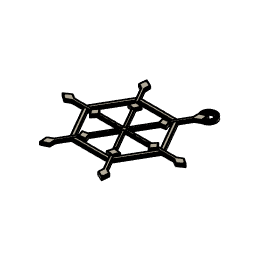
snowflake 4 (Autodesk Fusion 360 design; units mm, degrees)
Autodesk Fusion 360 part; units mm, degrees
note: some values were not read from the file. Chosen so that the rebuilt part matches the saved one: which bodies a step acts on.
(part 1 of 2)
sketch "Sketch1" plane through (0, 0, 0) normal (0, 0, 1) x (1, 0, 0)
  line L0 (-3.7004, 3.4114) -> (-1.9935, 3.4678)
  line L1 (-1.9935, 3.4678) -> (-1.0859, 4.9144)
  line L2 (-1.0859, 4.9144) -> (-2.4343, 6.3915)
  line L3 (-2.4343, 6.3915) -> (-20.127, 37.1684)
  line L4 (-20.127, 37.1684) -> (-21.9909, 36.0969)
  line L5 (-21.9909, 36.0969) -> (-4.2982, 5.32)
  line L6 (-4.2982, 5.32) -> (-3.7004, 3.4114)
  line L7 (-1.9935, 3.4678) -> (0, 0) construction
  dimension "d403" = 25
  dimension "d404" = 124
  dimension "d405" = 105.5
  dimension "d406" = 4
  dimension "d407" = 35.5
  dimension "d408" = 2.15
  dimension "d409" = 2
  dimension "d411" = 1.7068
  constraint coincident L7.end origin
  constraint symmetric L0 L1 L7
  constraint symmetric L2 L6 L7
  constraint symmetric L3 L5 L7
  constraint perpendicular L4 L5
  constraint perpendicular L3 L4
  measures "d403" angle of L2 L6
  measures "d404" angle of L0 L1
  measures "d405" angle of L1 L2
  measures "d406" distance of L0.end L7.end
  measures "d407" distance of L2.end L3.end
  measures "d408" distance of L3 L5
  measures "d409" distance of L1.end L2.end
  measures "d411" horizontal distance of L0.start L0.end
extrude "Extrude1" add sketch "Sketch1" along normal blind 5 makes body 1
pattern_circular "C-Pattern1" count 6 over 360 about axis through (0, 0, 1.75) along (0, 0, 1) of bodies 1 makes body 2 at (-18.5856, 1.1096, 1.6667) makes body 3 at (-14.3296, -26.8562, 1.6667) makes body 4 at (16.0934, -25.8379, 3.3333) makes body 5 at (18.5856, -1.1096, 1.6667) makes body 6 at (10.2538, 15.5408, 1.6667)
sketch "Sketch2" plane through (0, 0, 0) normal (0, 0, 1) x (1, 0, 0)
  line L0 (-31.5265, 40.9182) -> (-28.4205, 49.2257)
  line L1 (-28.4205, 49.2257) -> (-19.673, 47.7619)
  line L2 (-19.673, 47.7619) -> (-22.6772, 39.2781)
  line L3 (-22.6772, 39.2781) -> (-31.5265, 40.9182)
  line L4 (-28.4205, 49.2257) -> (-22.6772, 39.2781) construction
  line L5 (0, 1.75) -> (0, 22.5) construction
  line L6 (-20.127, 37.1684) -> (-21.9909, 36.0969) construction
  dimension "d416" = 30
  dimension "d417" = 3.1
  dimension "d418" = 99
  dimension "d419" = 80
  dimension "d420" = 9
  constraint coincident origin L4
  constraint symmetric L0 L1 L4
  constraint symmetric L2 L3 L4
  measures "d416" angle of L4 L5
  measures "d417" distance of L2.end L6
  measures "d418" angle of L2 L3
  measures "d419" angle of L1 L2
  measures "d420" distance of L1.end L2.end
extrude "Extrude2" add sketch "Sketch2" along normal up to surface (5 mm away) separate body makes body 7
pattern_circular "C-Pattern2" count 6 over 360 about axis through (0, 0, 1.75) along (0, 0, 1) of bodies 7 makes body 8 at (-51.1316, 2.2812, 0) makes body 9 at (-27.5414, -43.1407, 0) makes body 10 at (23.5902, -45.4219, 0) makes body 11 at (51.1316, -2.2812, 0) makes body 12 at (27.5414, 43.1407, 0)
sketch "Sketch3" plane through (0, 0, 0) normal (0, 0, 1) x (1, 0, 0)
  line L0 (-31.1618, 51.3738) -> (-29.6618, 51.3757)
  line L1 (-29.6618, 51.3757) -> (-28.9101, 52.6738)
  line L2 (-28.9101, 52.6738) -> (-43.4101, 77.7885)
  line L3 (-43.4101, 77.7885) -> (-43.4101, 86.9885)
  line L4 (-43.4101, 86.9885) -> (-50.3625, 90.2305)
  line L5 (-50.3625, 90.2305) -> (-52.9606, 88.7305)
  line L6 (-52.9606, 88.7305) -> (-53.6292, 81.0885)
  line L7 (-53.6292, 81.0885) -> (-45.6618, 76.4885)
  line L8 (-45.6618, 76.4885) -> (-31.1618, 51.3738)
  line L9 (-29.6618, 51.3757) -> (-51.6616, 89.4805) construction
  line L10 (0, 1.75) -> (0, 22.5) construction
  point P0 (-28.4205, 49.2257)
  dimension "d425" = 30
  dimension "d427" = 2.6
  dimension "d428" = 1.5
  dimension "d429" = 2.4826
  dimension "d430" = 60
  dimension "d431" = 70
  dimension "d432" = 3
  dimension "d433" = 9.2
  dimension "d434" = 29
  constraint midpoint L5 L9.end
  constraint coincident origin L9
  constraint symmetric L2 L8 L9
  constraint symmetric L0 L1 L9
  constraint symmetric L3 L7 L9
  constraint symmetric L4 L6 L9
  constraint perpendicular L5 L9
  constraint parallel L2 L8
  measures "d425" angle of L9 L10
  measures "d427" distance of L2 L8
  measures "d428" distance of L0.end L1.end
  measures "d429" distance of L0.end P0
  measures "d430" angle of L3 L7
  measures "d431" angle of L4 L6
  measures "d432" distance of L4.end L5.end
  measures "d433" distance of L2.end L3.end
  measures "d434" distance of L1.end L2.end
extrude "Extrude3" add sketch "Sketch3" along normal up to surface (5 mm away) separate body makes body 13
pattern_circular "C-Pattern3" count 6 over 360 about axis through (0, 0, 1.75) along (0, 0, 1) of bodies 13 makes body 14 at (-94.3835, 0.4333, 0) makes body 15 at (-47.567, -81.5218, 0) makes body 16 at (46.8165, -81.9552, 0) makes body 17 at (94.3835, -0.4333, 0) makes body 18 at (47.567, 81.5218, 0)
sketch "Sketch4" plane through (0, 0, 0) normal (0, 0, 1) x (1, 0, 0)
  line L0 (-3.7004, 3.4114) -> (-4.2982, 5.32)
  line L1 (-4.2982, 5.32) -> (-21.9909, 36.0969)
  line L2 (-21.9909, 36.0969) -> (-20.127, 37.1684)
  line L3 (-20.127, 37.1684) -> (-2.4343, 6.3915)
  line L4 (-2.4343, 6.3915) -> (-1.0859, 4.9144)
  line L5 (-1.0859, 4.9144) -> (-1.9935, 3.4678)
  line L6 (-1.9935, 3.4678) -> (-3.7004, 3.4114)
  line L7 (-19.673, 47.7619) -> (-22.6772, 39.2781)
  line L8 (-22.6772, 39.2781) -> (-31.5265, 40.9182)
  line L9 (-31.5265, 40.9182) -> (-28.4205, 49.2257)
  line L10 (-28.4205, 49.2257) -> (-19.673, 47.7619)
  line L11 (-31.1618, 51.3738) -> (-45.6618, 76.4885)
  line L12 (-45.6618, 76.4885) -> (-53.6292, 81.0885)
  line L13 (-53.6292, 81.0885) -> (-52.9606, 88.7305)
  line L14 (-52.9606, 88.7305) -> (-50.3625, 90.2305)
  line L15 (-50.3625, 90.2305) -> (-43.4101, 86.9885)
  line L16 (-43.4101, 86.9885) -> (-43.4101, 77.7885)
  line L17 (-43.4101, 77.7885) -> (-28.9101, 52.6738)
  line L18 (-28.9101, 52.6738) -> (-29.6618, 51.3757)
  line L19 (-29.6618, 51.3757) -> (-31.1618, 51.3738)
  line L20 (-19.5741, 39.2164) -> (-1.2157, 7.2815)
  line L21 (-1.2157, 7.2815) -> (0.791, 5.0833)
  line L22 (0.791, 5.0833) -> (-1.1469, 1.995)
  line L23 (-1.1469, 1.995) -> (-4.7908, 1.8745)
  line L24 (-4.7908, 1.8745) -> (-5.6805, 4.7148)
  line L25 (-5.6805, 4.7148) -> (-24.0389, 36.6497)
  line L26 (-24.0389, 36.6497) -> (-19.5741, 39.2164)
  line L27 (-33.5576, 39.7691) -> (-29.3924, 50.9092)
  line L28 (-29.3924, 50.9092) -> (-17.6623, 48.9462)
  line L29 (-17.6623, 48.9462) -> (-21.6909, 37.5697)
  line L30 (-21.6909, 37.5697) -> (-33.5576, 39.7691)
  line L31 (-28.7964, 49.8768) -> (-32.0271, 49.8726)
  line L32 (-32.0271, 49.8726) -> (-46.7598, 75.3904)
  line L33 (-46.7598, 75.3904) -> (-55.2068, 80.2673)
  line L34 (-55.2068, 80.2673) -> (-54.3868, 89.6391)
  line L35 (-54.3868, 89.6391) -> (-50.4363, 91.9199)
  line L36 (-50.4363, 91.9199) -> (-41.9101, 87.9441)
  line L37 (-41.9101, 87.9441) -> (-41.9101, 78.1904)
  line L38 (-41.9101, 78.1904) -> (-27.1774, 52.6726)
  line L39 (-27.1774, 52.6726) -> (-28.7964, 49.8768)
  line L40 (-54.3868, 89.6391) -> (-54.0403, 93.6005)
  line L41 (-54.0403, 93.6005) -> (-50.4363, 91.9199)
  line L42 (-27.1774, 52.6726) -> (-25.8135, 50.3103)
  line L43 (-32.0271, 49.8726) -> (-30.6632, 47.5103)
  line L44 (-19.5741, 39.2164) -> (-20.5232, 40.8673)
  line L45 (-24.0389, 36.6497) -> (-24.9109, 38.1665)
  dimension "d439" = -1.5
  dimension "d440" = -1.5
  dimension "d441" = -1.5
  constraint parallel L34 L40
  constraint collinear L36 L41
  constraint coincident L28 L42.end
  constraint parallel L38 L42
  constraint coincident L27 L43.end
  constraint parallel L32 L43
  constraint coincident L29 L44.end
  constraint perpendicular L26 L44
  constraint coincident L30 L45.end
  constraint perpendicular L26 L45
  measures "d441" distance of L19
extrude "Extrude4" add sketch "Sketch4" along normal up to surface (5 mm away) separate body makes body 19
pattern_circular "C-Pattern4" count 6 over 360 about axis through (0, 0, 1.75) along (0, 0, 1) of bodies 19 makes body 20 at (-105.9089, 0, 0) makes body 21 at (-52.9545, -91.7198, 0) makes body 22 at (52.9545, -91.7198, 0) makes body 23 at (105.9089, 0, 0) makes body 24 at (52.9545, 91.7198, 0)
combine "Combine1" operation add target body 19 tool bodies 21 24 22 23 20
sketch "Sketch5" plane through (0, 0, 0) normal (0, 0, 1) x (1, 0, 0)
  line L0 (-5.1366, 2.9784) -> (-5.6805, 4.7148)
  line L1 (-5.6805, 4.7148) -> (-24.9109, 38.1665)
  line L2 (-24.9109, 38.1665) -> (-33.5576, 39.7691)
  line L3 (-33.5576, 39.7691) -> (-30.6632, 47.5103)
  line L4 (-30.6632, 47.5103) -> (-46.7598, 75.3904)
  line L5 (-46.7598, 75.3904) -> (-55.2068, 80.2673)
  line L6 (-55.2068, 80.2673) -> (-54.0403, 93.6005)
  line L7 (-54.0403, 93.6005) -> (-41.9101, 87.9441)
  line L8 (-41.9101, 87.9441) -> (-41.9101, 78.1904)
  line L9 (-41.9101, 78.1904) -> (-25.8135, 50.3103)
  line L10 (-25.8135, 50.3103) -> (-17.6623, 48.9462)
  line L11 (-17.6623, 48.9462) -> (-20.5232, 40.8673)
  line L12 (-20.5232, 40.8673) -> (-1.2157, 7.2815)
  line L13 (-1.2157, 7.2815) -> (0.0111, 5.9377)
  line L14 (0.0111, 5.9377) -> (1.2429, 7.2769)
  line L15 (1.2429, 7.2769) -> (20.5977, 40.6567)
  line L16 (20.5977, 40.6567) -> (17.6623, 48.9462)
  line L17 (17.6623, 48.9462) -> (25.8135, 50.3103)
  line L18 (25.8135, 50.3103) -> (41.9101, 78.1904)
  line L19 (41.9101, 78.1904) -> (41.9101, 87.9441)
  line L20 (41.9101, 87.9441) -> (54.0403, 93.6005)
  line L21 (54.0403, 93.6005) -> (55.2068, 80.2673)
  line L22 (55.2068, 80.2673) -> (46.7598, 75.3904)
  line L23 (46.7598, 75.3904) -> (30.6632, 47.5103)
  line L24 (30.6632, 47.5103) -> (33.5576, 39.7691)
  line L25 (33.5576, 39.7691) -> (25.1306, 38.2072)
  line L26 (25.1306, 38.2072) -> (5.6981, 4.6936)
  line L27 (5.6981, 4.6936) -> (5.1477, 2.9592)
  line L28 (5.1477, 2.9592) -> (6.9234, 2.5621)
  line L29 (6.9234, 2.5621) -> (45.5086, 2.4902)
  line L30 (45.5086, 2.4902) -> (51.2198, 9.1772)
  line L31 (51.2198, 9.1772) -> (56.4767, 2.8)
  line L32 (56.4767, 2.8) -> (88.6699, 2.8)
  line L33 (88.6699, 2.8) -> (97.1169, 7.6768)
  line L34 (97.1169, 7.6768) -> (108.0805, 0)
  line L35 (108.0805, 0) -> (97.1169, -7.6768)
  line L36 (97.1169, -7.6768) -> (88.6699, -2.8)
  line L37 (88.6699, -2.8) -> (56.4767, -2.8)
  line L38 (56.4767, -2.8) -> (51.2198, -9.1772)
  line L39 (51.2198, -9.1772) -> (45.6537, -2.6601)
  line L40 (45.6537, -2.6601) -> (6.9138, -2.5879)
  line L41 (6.9138, -2.5879) -> (5.1366, -2.9784)
  line L42 (5.1366, -2.9784) -> (5.6805, -4.7148)
  line L43 (5.6805, -4.7148) -> (24.9109, -38.1665)
  line L44 (24.9109, -38.1665) -> (33.5576, -39.7691)
  line L45 (33.5576, -39.7691) -> (30.6632, -47.5103)
  line L46 (30.6632, -47.5103) -> (46.7598, -75.3904)
  line L47 (46.7598, -75.3904) -> (55.2068, -80.2673)
  line L48 (55.2068, -80.2673) -> (54.0403, -93.6005)
  line L49 (54.0403, -93.6005) -> (41.9101, -87.9441)
  line L50 (41.9101, -87.9441) -> (41.9101, -78.1904)
  line L51 (41.9101, -78.1904) -> (25.8135, -50.3103)
  line L52 (25.8135, -50.3103) -> (17.6623, -48.9462)
  line L53 (17.6623, -48.9462) -> (20.5232, -40.8673)
  line L54 (20.5232, -40.8673) -> (1.2157, -7.2815)
  line L55 (1.2157, -7.2815) -> (-0.0111, -5.9377)
  line L56 (-0.0111, -5.9377) -> (-1.2429, -7.2769)
  line L57 (-1.2429, -7.2769) -> (-20.5977, -40.6567)
  line L58 (-20.5977, -40.6567) -> (-17.6623, -48.9462)
  line L59 (-17.6623, -48.9462) -> (-25.8135, -50.3103)
  line L60 (-25.8135, -50.3103) -> (-41.9101, -78.1904)
  line L61 (-41.9101, -78.1904) -> (-41.9101, -87.9441)
  line L62 (-41.9101, -87.9441) -> (-54.0403, -93.6005)
  line L63 (-54.0403, -93.6005) -> (-55.2068, -80.2673)
  line L64 (-55.2068, -80.2673) -> (-46.7598, -75.3904)
  line L65 (-46.7598, -75.3904) -> (-30.6632, -47.5103)
  line L66 (-30.6632, -47.5103) -> (-33.5576, -39.7691)
  line L67 (-33.5576, -39.7691) -> (-25.1306, -38.2072)
  line L68 (-25.1306, -38.2072) -> (-5.6981, -4.6936)
  line L69 (-5.6981, -4.6936) -> (-5.1477, -2.9592)
  line L70 (-5.1477, -2.9592) -> (-6.9234, -2.5621)
  line L71 (-6.9234, -2.5621) -> (-45.5086, -2.4902)
  line L72 (-45.5086, -2.4902) -> (-51.2198, -9.1772)
  line L73 (-51.2198, -9.1772) -> (-56.4767, -2.8)
  line L74 (-56.4767, -2.8) -> (-88.6699, -2.8)
  line L75 (-88.6699, -2.8) -> (-97.1169, -7.6768)
  line L76 (-97.1169, -7.6768) -> (-108.0805, 0)
  line L77 (-108.0805, 0) -> (-97.1169, 7.6768)
  line L78 (-97.1169, 7.6768) -> (-88.6699, 2.8)
  line L79 (-88.6699, 2.8) -> (-56.4767, 2.8)
  line L80 (-56.4767, 2.8) -> (-51.2198, 9.1772)
  line L81 (-51.2198, 9.1772) -> (-45.6537, 2.6601)
  line L82 (-45.6537, 2.6601) -> (-6.9138, 2.5879)
  line L83 (-6.9138, 2.5879) -> (-5.1366, 2.9784)
  line L84 (-4, 0.0075) -> (-4.7989, 1.5168)
  line L85 (-4.7989, 1.5168) -> (-6.7523, 1.0876)
  line L86 (-6.7523, 1.0876) -> (-42.2523, 1.1537)
  line L87 (-42.2523, 1.1537) -> (-42.2563, -0.9962)
  line L88 (-42.2563, -0.9962) -> (-6.7563, -1.0624)
  line L89 (-6.7563, -1.0624) -> (-4.8046, -1.4989)
  line L90 (-4.8046, -1.4989) -> (-4, 0.0075)
  line L91 (-56.8409, 0) -> (-51.1995, -6.8437)
  line L92 (-51.1995, -6.8437) -> (-45.3544, 0)
  line L93 (-45.3544, 0) -> (-51.1995, 6.8437)
  line L94 (-51.1995, 6.8437) -> (-56.8409, 0)
  line L95 (-59.3235, 0) -> (-60.0719, 1.3)
  line L96 (-60.0719, 1.3) -> (-89.0719, 1.3)
  line L97 (-89.0719, 1.3) -> (-97.0393, 5.9)
  line L98 (-97.0393, 5.9) -> (-103.3231, 1.5)
  line L99 (-103.3231, 1.5) -> (-103.3231, -1.5)
  line L100 (-103.3231, -1.5) -> (-97.0393, -5.9)
  line L101 (-97.0393, -5.9) -> (-89.0719, -1.3)
  line L102 (-89.0719, -1.3) -> (-60.0719, -1.3)
  line L103 (-60.0719, -1.3) -> (-59.3235, 0)
  line L104 (-1.9935, 3.4678) -> (-1.0859, 4.9144)
  line L105 (-1.0859, 4.9144) -> (-2.4343, 6.3915)
  line L106 (-2.4343, 6.3915) -> (-20.127, 37.1684)
  line L107 (-20.127, 37.1684) -> (-21.9909, 36.0969)
  line L108 (-21.9909, 36.0969) -> (-4.2982, 5.32)
  line L109 (-4.2982, 5.32) -> (-3.7004, 3.4114)
  line L110 (-3.7004, 3.4114) -> (-1.9935, 3.4678)
  line L111 (-28.4205, 49.2257) -> (-31.5265, 40.9182)
  line L112 (-31.5265, 40.9182) -> (-22.6772, 39.2781)
  line L113 (-22.6772, 39.2781) -> (-19.673, 47.7619)
  line L114 (-19.673, 47.7619) -> (-28.4205, 49.2257)
  line L115 (-29.6618, 51.3757) -> (-28.9101, 52.6738)
  line L116 (-28.9101, 52.6738) -> (-43.4101, 77.7885)
  line L117 (-43.4101, 77.7885) -> (-43.4101, 86.9885)
  line L118 (-43.4101, 86.9885) -> (-50.3625, 90.2305)
  line L119 (-50.3625, 90.2305) -> (-52.9606, 88.7305)
  line L120 (-52.9606, 88.7305) -> (-53.6292, 81.0885)
  line L121 (-53.6292, 81.0885) -> (-45.6618, 76.4885)
  line L122 (-45.6618, 76.4885) -> (-31.1618, 51.3738)
  line L123 (-31.1618, 51.3738) -> (-29.6618, 51.3757)
  line L124 (2.0065, 3.4604) -> (3.7131, 3.3976)
  line L125 (3.7131, 3.3976) -> (4.318, 5.3039)
  line L126 (4.318, 5.3039) -> (22.1253, 36.0147)
  line L127 (22.1253, 36.0147) -> (20.2654, 37.0931)
  line L128 (20.2654, 37.0931) -> (2.4581, 6.3824)
  line L129 (2.4581, 6.3824) -> (1.1042, 4.9103)
  line L130 (1.1042, 4.9103) -> (2.0065, 3.4604)
  line L131 (28.4205, 49.2257) -> (19.673, 47.7619)
  line L132 (19.673, 47.7619) -> (22.6772, 39.2781)
  line L133 (22.6772, 39.2781) -> (31.5265, 40.9182)
  line L134 (31.5265, 40.9182) -> (28.4205, 49.2257)
  line L135 (29.6618, 51.3757) -> (31.1618, 51.3738)
  line L136 (31.1618, 51.3738) -> (45.6618, 76.4885)
  line L137 (45.6618, 76.4885) -> (53.6292, 81.0885)
  line L138 (53.6292, 81.0885) -> (52.9606, 88.7305)
  line L139 (52.9606, 88.7305) -> (50.3625, 90.2305)
  line L140 (50.3625, 90.2305) -> (43.4101, 86.9885)
  line L141 (43.4101, 86.9885) -> (43.4101, 77.7885)
  line L142 (43.4101, 77.7885) -> (28.9101, 52.6738)
  line L143 (28.9101, 52.6738) -> (29.6618, 51.3757)
  line L144 (59.3235, 0) -> (60.0719, -1.3)
  line L145 (60.0719, -1.3) -> (89.0719, -1.3)
  line L146 (89.0719, -1.3) -> (97.0393, -5.9)
  line L147 (97.0393, -5.9) -> (103.3231, -1.5)
  line L148 (103.3231, -1.5) -> (103.3231, 1.5)
  line L149 (103.3231, 1.5) -> (97.0393, 5.9)
  line L150 (97.0393, 5.9) -> (89.0719, 1.3)
  line L151 (89.0719, 1.3) -> (60.0719, 1.3)
  line L152 (60.0719, 1.3) -> (59.3235, 0)
  line L153 (56.8409, 0) -> (51.1995, 6.8437)
  line L154 (51.1995, 6.8437) -> (45.3544, 0)
  line L155 (45.3544, 0) -> (51.1995, -6.8437)
  line L156 (51.1995, -6.8437) -> (56.8409, 0)
  line L157 (4, -0.0075) -> (4.7989, -1.5168)
  line L158 (4.7989, -1.5168) -> (6.7523, -1.0876)
  line L159 (6.7523, -1.0876) -> (42.2523, -1.1537)
  line L160 (42.2523, -1.1537) -> (42.2563, 0.9962)
  line L161 (42.2563, 0.9962) -> (6.7563, 1.0624)
  line L162 (6.7563, 1.0624) -> (4.8046, 1.4989)
  line L163 (4.8046, 1.4989) -> (4, -0.0075)
  line L164 (29.6618, -51.3757) -> (28.9101, -52.6738)
  line L165 (28.9101, -52.6738) -> (43.4101, -77.7885)
  line L166 (43.4101, -77.7885) -> (43.4101, -86.9885)
  line L167 (43.4101, -86.9885) -> (50.3625, -90.2305)
  line L168 (50.3625, -90.2305) -> (52.9606, -88.7305)
  line L169 (52.9606, -88.7305) -> (53.6292, -81.0885)
  line L170 (53.6292, -81.0885) -> (45.6618, -76.4885)
  line L171 (45.6618, -76.4885) -> (31.1618, -51.3738)
  line L172 (31.1618, -51.3738) -> (29.6618, -51.3757)
  line L173 (28.4205, -49.2257) -> (31.5265, -40.9182)
  line L174 (31.5265, -40.9182) -> (22.6772, -39.2781)
  line L175 (22.6772, -39.2781) -> (19.673, -47.7619)
  line L176 (19.673, -47.7619) -> (28.4205, -49.2257)
  line L177 (1.9935, -3.4678) -> (1.0859, -4.9144)
  line L178 (1.0859, -4.9144) -> (2.4343, -6.3915)
  line L179 (2.4343, -6.3915) -> (20.127, -37.1684)
  line L180 (20.127, -37.1684) -> (21.9909, -36.0969)
  line L181 (21.9909, -36.0969) -> (4.2982, -5.32)
  line L182 (4.2982, -5.32) -> (3.7004, -3.4114)
  line L183 (3.7004, -3.4114) -> (1.9935, -3.4678)
  line L184 (-29.6618, -51.3757) -> (-31.1618, -51.3738)
  line L185 (-31.1618, -51.3738) -> (-45.6618, -76.4885)
  line L186 (-45.6618, -76.4885) -> (-53.6292, -81.0885)
  line L187 (-53.6292, -81.0885) -> (-52.9606, -88.7305)
  line L188 (-52.9606, -88.7305) -> (-50.3625, -90.2305)
  line L189 (-50.3625, -90.2305) -> (-43.4101, -86.9885)
  line L190 (-43.4101, -86.9885) -> (-43.4101, -77.7885)
  line L191 (-43.4101, -77.7885) -> (-28.9101, -52.6738)
  line L192 (-28.9101, -52.6738) -> (-29.6618, -51.3757)
  line L193 (-28.4205, -49.2257) -> (-19.673, -47.7619)
  line L194 (-19.673, -47.7619) -> (-22.6772, -39.2781)
  line L195 (-22.6772, -39.2781) -> (-31.5265, -40.9182)
  line L196 (-31.5265, -40.9182) -> (-28.4205, -49.2257)
  line L197 (-2.0065, -3.4604) -> (-3.7131, -3.3976)
  line L198 (-3.7131, -3.3976) -> (-4.318, -5.3039)
  line L199 (-4.318, -5.3039) -> (-22.1253, -36.0147)
  line L200 (-22.1253, -36.0147) -> (-20.2654, -37.0931)
  line L201 (-20.2654, -37.0931) -> (-2.4581, -6.3824)
  line L202 (-2.4581, -6.3824) -> (-1.1042, -4.9103)
  line L203 (-1.1042, -4.9103) -> (-2.0065, -3.4604)
  line L204 (-3.3169, 1.9233) -> (-2.3011, 0.0043)
  line L205 (-2.3011, 0.0043) -> (-3.324, -1.9109)
  line L206 (-3.324, -1.9109) -> (-1.1543, -1.9907)
  line L207 (-1.1543, -1.9907) -> (-0.0071, -3.8341)
  line L208 (-0.0071, -3.8341) -> (1.1469, -1.995)
  line L209 (1.1469, -1.995) -> (3.3169, -1.9233)
  line L210 (3.3169, -1.9233) -> (2.3011, -0.0043)
  line L211 (2.3011, -0.0043) -> (3.324, 1.9109)
  line L212 (3.324, 1.9109) -> (1.1543, 1.9907)
  line L213 (1.1543, 1.9907) -> (0.0071, 3.8341)
  line L214 (0.0071, 3.8341) -> (-1.1469, 1.995)
  line L215 (-1.1469, 1.995) -> (-3.3169, 1.9233)
extrude "Extrude5" add sketch "Sketch5" along normal up to surface (5 mm away) separate body contours L204 L205 L206 L207 L208 L209 L210 L211 L212 L213 L214 L215 makes body 25
sketch "Sketch6" plane through (0, 0, 0) normal (0, 0, 1) x (1, 0, 0)
  line L0 (-5.1366, 2.9784) -> (-5.6805, 4.7148)
  line L1 (-5.6805, 4.7148) -> (-24.9109, 38.1665)
  line L2 (-24.9109, 38.1665) -> (-33.5576, 39.7691)
  line L3 (-33.5576, 39.7691) -> (-30.6632, 47.5103)
  line L4 (-30.6632, 47.5103) -> (-46.7598, 75.3904)
  line L5 (-46.7598, 75.3904) -> (-55.2068, 80.2673)
  line L6 (-55.2068, 80.2673) -> (-54.0403, 93.6005)
  line L7 (-54.0403, 93.6005) -> (-41.9101, 87.9441)
  line L8 (-41.9101, 87.9441) -> (-41.9101, 78.1904)
  line L9 (-41.9101, 78.1904) -> (-25.8135, 50.3103)
  line L10 (-25.8135, 50.3103) -> (-17.6623, 48.9462)
  line L11 (-17.6623, 48.9462) -> (-20.5232, 40.8673)
  line L12 (-20.5232, 40.8673) -> (-1.2157, 7.2815)
  line L13 (-1.2157, 7.2815) -> (0.0111, 5.9377)
  line L14 (0.0111, 5.9377) -> (1.2429, 7.2769)
  line L15 (1.2429, 7.2769) -> (20.5977, 40.6567)
  line L16 (20.5977, 40.6567) -> (17.6623, 48.9462)
  line L17 (17.6623, 48.9462) -> (25.8135, 50.3103)
  line L18 (25.8135, 50.3103) -> (41.9101, 78.1904)
  line L19 (41.9101, 78.1904) -> (41.9101, 87.9441)
  line L20 (41.9101, 87.9441) -> (54.0403, 93.6005)
  line L21 (54.0403, 93.6005) -> (55.2068, 80.2673)
  line L22 (55.2068, 80.2673) -> (46.7598, 75.3904)
  line L23 (46.7598, 75.3904) -> (30.6632, 47.5103)
  line L24 (30.6632, 47.5103) -> (33.5576, 39.7691)
  line L25 (33.5576, 39.7691) -> (25.1306, 38.2072)
  line L26 (25.1306, 38.2072) -> (5.6981, 4.6936)
  line L27 (5.6981, 4.6936) -> (5.1477, 2.9592)
  line L28 (5.1477, 2.9592) -> (6.9234, 2.5621)
  line L29 (6.9234, 2.5621) -> (45.5086, 2.4902)
  line L30 (45.5086, 2.4902) -> (51.2198, 9.1772)
  line L31 (51.2198, 9.1772) -> (56.4767, 2.8)
  line L32 (56.4767, 2.8) -> (88.6699, 2.8)
  line L33 (88.6699, 2.8) -> (97.1169, 7.6768)
  line L34 (97.1169, 7.6768) -> (108.0805, 0)
  line L35 (108.0805, 0) -> (97.1169, -7.6768)
  line L36 (97.1169, -7.6768) -> (88.6699, -2.8)
  line L37 (88.6699, -2.8) -> (56.4767, -2.8)
  line L38 (56.4767, -2.8) -> (51.2198, -9.1772)
  line L39 (51.2198, -9.1772) -> (45.6537, -2.6601)
  line L40 (45.6537, -2.6601) -> (6.9138, -2.5879)
  line L41 (6.9138, -2.5879) -> (5.1366, -2.9784)
  line L42 (5.1366, -2.9784) -> (5.6805, -4.7148)
  line L43 (5.6805, -4.7148) -> (24.9109, -38.1665)
  line L44 (24.9109, -38.1665) -> (33.5576, -39.7691)
  line L45 (33.5576, -39.7691) -> (30.6632, -47.5103)
  line L46 (30.6632, -47.5103) -> (46.7598, -75.3904)
  line L47 (46.7598, -75.3904) -> (55.2068, -80.2673)
  line L48 (55.2068, -80.2673) -> (54.0403, -93.6005)
  line L49 (54.0403, -93.6005) -> (41.9101, -87.9441)
  line L50 (41.9101, -87.9441) -> (41.9101, -78.1904)
  line L51 (41.9101, -78.1904) -> (25.8135, -50.3103)
  line L52 (25.8135, -50.3103) -> (17.6623, -48.9462)
  line L53 (17.6623, -48.9462) -> (20.5232, -40.8673)
  line L54 (20.5232, -40.8673) -> (1.2157, -7.2815)
  line L55 (1.2157, -7.2815) -> (-0.0111, -5.9377)
  line L56 (-0.0111, -5.9377) -> (-1.2429, -7.2769)
  line L57 (-1.2429, -7.2769) -> (-20.5977, -40.6567)
  line L58 (-20.5977, -40.6567) -> (-17.6623, -48.9462)
  line L59 (-17.6623, -48.9462) -> (-25.8135, -50.3103)
  line L60 (-25.8135, -50.3103) -> (-41.9101, -78.1904)
  line L61 (-41.9101, -78.1904) -> (-41.9101, -87.9441)
  line L62 (-41.9101, -87.9441) -> (-54.0403, -93.6005)
  line L63 (-54.0403, -93.6005) -> (-55.2068, -80.2673)
  line L64 (-55.2068, -80.2673) -> (-46.7598, -75.3904)
  line L65 (-46.7598, -75.3904) -> (-30.6632, -47.5103)
  line L66 (-30.6632, -47.5103) -> (-33.5576, -39.7691)
  line L67 (-33.5576, -39.7691) -> (-25.1306, -38.2072)
  line L68 (-25.1306, -38.2072) -> (-5.6981, -4.6936)
  line L69 (-5.6981, -4.6936) -> (-5.1477, -2.9592)
  line L70 (-5.1477, -2.9592) -> (-6.9234, -2.5621)
  line L71 (-6.9234, -2.5621) -> (-45.5086, -2.4902)
  line L72 (-45.5086, -2.4902) -> (-51.2198, -9.1772)
  line L73 (-51.2198, -9.1772) -> (-56.4767, -2.8)
  line L74 (-56.4767, -2.8) -> (-88.6699, -2.8)
  line L75 (-88.6699, -2.8) -> (-97.1169, -7.6768)
  line L76 (-97.1169, -7.6768) -> (-108.0805, 0)
  line L77 (-108.0805, 0) -> (-97.1169, 7.6768)
  line L78 (-97.1169, 7.6768) -> (-88.6699, 2.8)
  line L79 (-88.6699, 2.8) -> (-56.4767, 2.8)
  line L80 (-56.4767, 2.8) -> (-51.2198, 9.1772)
  line L81 (-51.2198, 9.1772) -> (-45.6537, 2.6601)
  line L82 (-45.6537, 2.6601) -> (-6.9138, 2.5879)
  line L83 (-6.9138, 2.5879) -> (-5.1366, 2.9784)
  line L84 (-4, 0.0075) -> (-4.7989, 1.5168)
  line L85 (-4.7989, 1.5168) -> (-6.7523, 1.0876)
  line L86 (-6.7523, 1.0876) -> (-42.2523, 1.1537)
  line L87 (-42.2523, 1.1537) -> (-42.2563, -0.9962)
  line L88 (-42.2563, -0.9962) -> (-6.7563, -1.0624)
  line L89 (-6.7563, -1.0624) -> (-4.8046, -1.4989)
  line L90 (-4.8046, -1.4989) -> (-4, 0.0075)
  line L91 (-56.8409, 0) -> (-51.1995, -6.8437)
  line L92 (-51.1995, -6.8437) -> (-45.3544, 0)
  line L93 (-45.3544, 0) -> (-51.1995, 6.8437)
  line L94 (-51.1995, 6.8437) -> (-56.8409, 0)
  line L95 (-59.3235, 0) -> (-60.0719, 1.3)
  line L96 (-60.0719, 1.3) -> (-89.0719, 1.3)
  line L97 (-89.0719, 1.3) -> (-97.0393, 5.9)
  line L98 (-97.0393, 5.9) -> (-103.3231, 1.5)
  line L99 (-103.3231, 1.5) -> (-103.3231, -1.5)
  line L100 (-103.3231, -1.5) -> (-97.0393, -5.9)
  line L101 (-97.0393, -5.9) -> (-89.0719, -1.3)
  line L102 (-89.0719, -1.3) -> (-60.0719, -1.3)
  line L103 (-60.0719, -1.3) -> (-59.3235, 0)
  line L104 (-1.9935, 3.4678) -> (-1.0859, 4.9144)
  line L105 (-1.0859, 4.9144) -> (-2.4343, 6.3915)
  line L106 (-2.4343, 6.3915) -> (-20.127, 37.1684)
  line L107 (-20.127, 37.1684) -> (-21.9909, 36.0969)
  line L108 (-21.9909, 36.0969) -> (-4.2982, 5.32)
  line L109 (-4.2982, 5.32) -> (-3.7004, 3.4114)
  line L110 (-3.7004, 3.4114) -> (-1.9935, 3.4678)
  line L111 (-28.4205, 49.2257) -> (-31.5265, 40.9182)
  line L112 (-31.5265, 40.9182) -> (-22.6772, 39.2781)
  line L113 (-22.6772, 39.2781) -> (-19.673, 47.7619)
  line L114 (-19.673, 47.7619) -> (-28.4205, 49.2257)
  line L115 (-29.6618, 51.3757) -> (-28.9101, 52.6738)
  line L116 (-28.9101, 52.6738) -> (-43.4101, 77.7885)
  line L117 (-43.4101, 77.7885) -> (-43.4101, 86.9885)
  line L118 (-43.4101, 86.9885) -> (-50.3625, 90.2305)
  line L119 (-50.3625, 90.2305) -> (-52.9606, 88.7305)
  line L120 (-52.9606, 88.7305) -> (-53.6292, 81.0885)
  line L121 (-53.6292, 81.0885) -> (-45.6618, 76.4885)
  line L122 (-45.6618, 76.4885) -> (-31.1618, 51.3738)
  line L123 (-31.1618, 51.3738) -> (-29.6618, 51.3757)
  line L124 (2.0065, 3.4604) -> (3.7131, 3.3976)
  line L125 (3.7131, 3.3976) -> (4.318, 5.3039)
  line L126 (4.318, 5.3039) -> (22.1253, 36.0147)
  line L127 (22.1253, 36.0147) -> (20.2654, 37.0931)
  line L128 (20.2654, 37.0931) -> (2.4581, 6.3824)
  line L129 (2.4581, 6.3824) -> (1.1042, 4.9103)
  line L130 (1.1042, 4.9103) -> (2.0065, 3.4604)
  line L131 (28.4205, 49.2257) -> (19.673, 47.7619)
  line L132 (19.673, 47.7619) -> (22.6772, 39.2781)
  line L133 (22.6772, 39.2781) -> (31.5265, 40.9182)
  line L134 (31.5265, 40.9182) -> (28.4205, 49.2257)
  line L135 (29.6618, 51.3757) -> (31.1618, 51.3738)
  line L136 (31.1618, 51.3738) -> (45.6618, 76.4885)
  line L137 (45.6618, 76.4885) -> (53.6292, 81.0885)
  line L138 (53.6292, 81.0885) -> (52.9606, 88.7305)
  line L139 (52.9606, 88.7305) -> (50.3625, 90.2305)
  line L140 (50.3625, 90.2305) -> (43.4101, 86.9885)
  line L141 (43.4101, 86.9885) -> (43.4101, 77.7885)
  line L142 (43.4101, 77.7885) -> (28.9101, 52.6738)
  line L143 (28.9101, 52.6738) -> (29.6618, 51.3757)
  line L144 (59.3235, 0) -> (60.0719, -1.3)
  line L145 (60.0719, -1.3) -> (89.0719, -1.3)
  line L146 (89.0719, -1.3) -> (97.0393, -5.9)
  line L147 (97.0393, -5.9) -> (103.3231, -1.5)
  line L148 (103.3231, -1.5) -> (103.3231, 1.5)
  line L149 (103.3231, 1.5) -> (97.0393, 5.9)
  line L150 (97.0393, 5.9) -> (89.0719, 1.3)
  line L151 (89.0719, 1.3) -> (60.0719, 1.3)
  line L152 (60.0719, 1.3) -> (59.3235, 0)
  line L153 (56.8409, 0) -> (51.1995, 6.8437)
  line L154 (51.1995, 6.8437) -> (45.3544, 0)
  line L155 (45.3544, 0) -> (51.1995, -6.8437)
  line L156 (51.1995, -6.8437) -> (56.8409, 0)
  line L157 (4, -0.0075) -> (4.7989, -1.5168)
  line L158 (4.7989, -1.5168) -> (6.7523, -1.0876)
  line L159 (6.7523, -1.0876) -> (42.2523, -1.1537)
  line L160 (42.2523, -1.1537) -> (42.2563, 0.9962)
  line L161 (42.2563, 0.9962) -> (6.7563, 1.0624)
  line L162 (6.7563, 1.0624) -> (4.8046, 1.4989)
  line L163 (4.8046, 1.4989) -> (4, -0.0075)
  line L164 (29.6618, -51.3757) -> (28.9101, -52.6738)
  line L165 (28.9101, -52.6738) -> (43.4101, -77.7885)
  line L166 (43.4101, -77.7885) -> (43.4101, -86.9885)
  line L167 (43.4101, -86.9885) -> (50.3625, -90.2305)
  line L168 (50.3625, -90.2305) -> (52.9606, -88.7305)
  line L169 (52.9606, -88.7305) -> (53.6292, -81.0885)
  line L170 (53.6292, -81.0885) -> (45.6618, -76.4885)
  line L171 (45.6618, -76.4885) -> (31.1618, -51.3738)
  line L172 (31.1618, -51.3738) -> (29.6618, -51.3757)
  line L173 (28.4205, -49.2257) -> (31.5265, -40.9182)
  line L174 (31.5265, -40.9182) -> (22.6772, -39.2781)
  line L175 (22.6772, -39.2781) -> (19.673, -47.7619)
  line L176 (19.673, -47.7619) -> (28.4205, -49.2257)
  line L177 (1.9935, -3.4678) -> (1.0859, -4.9144)
  line L178 (1.0859, -4.9144) -> (2.4343, -6.3915)
  line L179 (2.4343, -6.3915) -> (20.127, -37.1684)
  line L180 (20.127, -37.1684) -> (21.9909, -36.0969)
  line L181 (21.9909, -36.0969) -> (4.2982, -5.32)
  line L182 (4.2982, -5.32) -> (3.7004, -3.4114)
  line L183 (3.7004, -3.4114) -> (1.9935, -3.4678)
  line L184 (-29.6618, -51.3757) -> (-31.1618, -51.3738)
  line L185 (-31.1618, -51.3738) -> (-45.6618, -76.4885)
  line L186 (-45.6618, -76.4885) -> (-53.6292, -81.0885)
  line L187 (-53.6292, -81.0885) -> (-52.9606, -88.7305)
  line L188 (-52.9606, -88.7305) -> (-50.3625, -90.2305)
  line L189 (-50.3625, -90.2305) -> (-43.4101, -86.9885)
  line L190 (-43.4101, -86.9885) -> (-43.4101, -77.7885)
  line L191 (-43.4101, -77.7885) -> (-28.9101, -52.6738)
  line L192 (-28.9101, -52.6738) -> (-29.6618, -51.3757)
  line L193 (-28.4205, -49.2257) -> (-19.673, -47.7619)
  line L194 (-19.673, -47.7619) -> (-22.6772, -39.2781)
  line L195 (-22.6772, -39.2781) -> (-31.5265, -40.9182)
  line L196 (-31.5265, -40.9182) -> (-28.4205, -49.2257)
  line L197 (-2.0065, -3.4604) -> (-3.7131, -3.3976)
  line L198 (-3.7131, -3.3976) -> (-4.318, -5.3039)
  line L199 (-4.318, -5.3039) -> (-22.1253, -36.0147)
  line L200 (-22.1253, -36.0147) -> (-20.2654, -37.0931)
  line L201 (-20.2654, -37.0931) -> (-2.4581, -6.3824)
  line L202 (-2.4581, -6.3824) -> (-1.1042, -4.9103)
  line L203 (-1.1042, -4.9103) -> (-2.0065, -3.4604)
  line L204 (-3.3169, 1.9233) -> (-2.3011, 0.0043)
  line L205 (-2.3011, 0.0043) -> (-3.324, -1.9109)
  line L206 (-3.324, -1.9109) -> (-1.1543, -1.9907)
  line L207 (-1.1543, -1.9907) -> (-0.0071, -3.8341)
  line L208 (-0.0071, -3.8341) -> (1.1469, -1.995)
  line L209 (1.1469, -1.995) -> (3.3169, -1.9233)
  line L210 (3.3169, -1.9233) -> (2.3011, -0.0043)
  line L211 (2.3011, -0.0043) -> (3.324, 1.9109)
  line L212 (3.324, 1.9109) -> (1.1543, 1.9907)
  line L213 (1.1543, 1.9907) -> (0.0071, 3.8341)
  line L214 (0.0071, 3.8341) -> (-1.1469, 1.995)
  line L215 (-1.1469, 1.995) -> (-3.3169, 1.9233)
  line L216 (-28.7946, 55.4737) -> (28.7946, 55.4737)
  line L217 (30.7773, 58.9078) -> (-30.7773, 58.9078)
  constraint coincident L9 L216.start
  constraint coincident L18 L216.end
  constraint horizontal L216
  constraint coincident L18 L217.start
  constraint coincident L9 L217.end
  constraint parallel L216 L217
extrude "Extrude6" add sketch "Sketch6" along normal up to surface (5 mm away) separate body contours L9 L18 L216 L217 makes body 26
pattern_circular "C-Pattern5" count 6 over 360 about axis through (0, 0, 1.75) along (0, 0, 1) of bodies 26 makes body 27 at (-45.8861, 38.3385, 1.6667) makes body 28 at (-56.1452, -20.5693, 1.6667) makes body 29 at (-10.2591, -58.9078, 1.6667) makes body 30 at (45.8861, -38.3385, 1.6667) makes body 31 at (56.1452, 20.5693, 1.6667)
sketch "Sketch7" plane through (0, 0, 0) normal (0, 0, 1) x (1, 0, 0)
  line L0 (-30.7773, 58.9078) -> (30.7773, 58.9078)
  line L1 (30.7773, 58.9078) -> (28.7946, 55.4737)
  line L2 (28.7946, 55.4737) -> (-28.7946, 55.4737)
  line L3 (-28.7946, 55.4737) -> (-30.7773, 58.9078)
  line L4 (29.6606, 53.9737) -> (-29.6606, 53.9737)
  line L5 (-29.6606, 53.9737) -> (-33.3753, 60.4078)
  line L6 (-33.3753, 60.4078) -> (33.3753, 60.4078)
  line L7 (33.3753, 60.4078) -> (29.6606, 53.9737)
  line L8 (-5.1366, 2.9784) -> (-5.6805, 4.7148)
  line L9 (-5.6805, 4.7148) -> (-24.9109, 38.1665)
  line L10 (-24.9109, 38.1665) -> (-33.5576, 39.7691)
  line L11 (-33.5576, 39.7691) -> (-30.6632, 47.5103)
  line L12 (-30.6632, 47.5103) -> (-46.7598, 75.3904)
  line L13 (-46.7598, 75.3904) -> (-55.2068, 80.2673)
  line L14 (-55.2068, 80.2673) -> (-54.0403, 93.6005)
  line L15 (-54.0403, 93.6005) -> (-41.9101, 87.9441)
  line L16 (-41.9101, 87.9441) -> (-41.9101, 78.1904)
  line L17 (-41.9101, 78.1904) -> (-25.8135, 50.3103)
  line L18 (-25.8135, 50.3103) -> (-17.6623, 48.9462)
  line L19 (-17.6623, 48.9462) -> (-20.5232, 40.8673)
  line L20 (-20.5232, 40.8673) -> (-1.2157, 7.2815)
  line L21 (-1.2157, 7.2815) -> (0.0111, 5.9377)
  line L22 (0.0111, 5.9377) -> (1.2429, 7.2769)
  line L23 (1.2429, 7.2769) -> (20.5977, 40.6567)
  line L24 (20.5977, 40.6567) -> (17.6623, 48.9462)
  line L25 (17.6623, 48.9462) -> (25.8135, 50.3103)
  line L26 (25.8135, 50.3103) -> (41.9101, 78.1904)
  line L27 (41.9101, 78.1904) -> (41.9101, 87.9441)
  line L28 (41.9101, 87.9441) -> (54.0403, 93.6005)
  line L29 (54.0403, 93.6005) -> (55.2068, 80.2673)
  line L30 (55.2068, 80.2673) -> (46.7598, 75.3904)
  line L31 (46.7598, 75.3904) -> (30.6632, 47.5103)
  line L32 (30.6632, 47.5103) -> (33.5576, 39.7691)
  line L33 (33.5576, 39.7691) -> (25.1306, 38.2072)
  line L34 (25.1306, 38.2072) -> (5.6981, 4.6936)
  line L35 (5.6981, 4.6936) -> (5.1477, 2.9592)
  line L36 (5.1477, 2.9592) -> (6.9234, 2.5621)
  line L37 (6.9234, 2.5621) -> (45.5086, 2.4902)
  line L38 (45.5086, 2.4902) -> (51.2198, 9.1772)
  line L39 (51.2198, 9.1772) -> (56.4767, 2.8)
  line L40 (56.4767, 2.8) -> (88.6699, 2.8)
  line L41 (88.6699, 2.8) -> (97.1169, 7.6768)
  line L42 (97.1169, 7.6768) -> (108.0805, 0)
  line L43 (108.0805, 0) -> (97.1169, -7.6768)
  line L44 (97.1169, -7.6768) -> (88.6699, -2.8)
  line L45 (88.6699, -2.8) -> (56.4767, -2.8)
  line L46 (56.4767, -2.8) -> (51.2198, -9.1772)
  line L47 (51.2198, -9.1772) -> (45.6537, -2.6601)
  line L48 (45.6537, -2.6601) -> (6.9138, -2.5879)
  line L49 (6.9138, -2.5879) -> (5.1366, -2.9784)
  line L50 (5.1366, -2.9784) -> (5.6805, -4.7148)
  line L51 (5.6805, -4.7148) -> (24.9109, -38.1665)
  line L52 (24.9109, -38.1665) -> (33.5576, -39.7691)
  line L53 (33.5576, -39.7691) -> (30.6632, -47.5103)
  line L54 (30.6632, -47.5103) -> (46.7598, -75.3904)
  line L55 (46.7598, -75.3904) -> (55.2068, -80.2673)
  line L56 (55.2068, -80.2673) -> (54.0403, -93.6005)
  line L57 (54.0403, -93.6005) -> (41.9101, -87.9441)
  line L58 (41.9101, -87.9441) -> (41.9101, -78.1904)
  line L59 (41.9101, -78.1904) -> (25.8135, -50.3103)
  line L60 (25.8135, -50.3103) -> (17.6623, -48.9462)
  line L61 (17.6623, -48.9462) -> (20.5232, -40.8673)
  line L62 (20.5232, -40.8673) -> (1.2157, -7.2815)
  line L63 (1.2157, -7.2815) -> (-0.0111, -5.9377)
  line L64 (-0.0111, -5.9377) -> (-1.2429, -7.2769)
  line L65 (-1.2429, -7.2769) -> (-20.5977, -40.6567)
  line L66 (-20.5977, -40.6567) -> (-17.6623, -48.9462)
  line L67 (-17.6623, -48.9462) -> (-25.8135, -50.3103)
  line L68 (-25.8135, -50.3103) -> (-41.9101, -78.1904)
  line L69 (-41.9101, -78.1904) -> (-41.9101, -87.9441)
  line L70 (-41.9101, -87.9441) -> (-54.0403, -93.6005)
  line L71 (-54.0403, -93.6005) -> (-55.2068, -80.2673)
  line L72 (-55.2068, -80.2673) -> (-46.7598, -75.3904)
  line L73 (-46.7598, -75.3904) -> (-30.6632, -47.5103)
  line L74 (-30.6632, -47.5103) -> (-33.5576, -39.7691)
  line L75 (-33.5576, -39.7691) -> (-25.1306, -38.2072)
  line L76 (-25.1306, -38.2072) -> (-5.6981, -4.6936)
  line L77 (-5.6981, -4.6936) -> (-5.1477, -2.9592)
  line L78 (-5.1477, -2.9592) -> (-6.9234, -2.5621)
  line L79 (-6.9234, -2.5621) -> (-45.5086, -2.4902)
  line L80 (-45.5086, -2.4902) -> (-51.2198, -9.1772)
  line L81 (-51.2198, -9.1772) -> (-56.4767, -2.8)
  line L82 (-56.4767, -2.8) -> (-88.6699, -2.8)
  line L83 (-88.6699, -2.8) -> (-97.1169, -7.6768)
  line L84 (-97.1169, -7.6768) -> (-108.0805, 0)
  line L85 (-108.0805, 0) -> (-97.1169, 7.6768)
  line L86 (-97.1169, 7.6768) -> (-88.6699, 2.8)
  line L87 (-88.6699, 2.8) -> (-56.4767, 2.8)
  line L88 (-56.4767, 2.8) -> (-51.2198, 9.1772)
  line L89 (-51.2198, 9.1772) -> (-45.6537, 2.6601)
  line L90 (-45.6537, 2.6601) -> (-6.9138, 2.5879)
  line L91 (-6.9138, 2.5879) -> (-5.1366, 2.9784)
  line L92 (-4, 0.0075) -> (-4.7989, 1.5168)
  line L93 (-4.7989, 1.5168) -> (-6.7523, 1.0876)
  line L94 (-6.7523, 1.0876) -> (-42.2523, 1.1537)
  line L95 (-42.2523, 1.1537) -> (-42.2563, -0.9962)
  line L96 (-42.2563, -0.9962) -> (-6.7563, -1.0624)
  line L97 (-6.7563, -1.0624) -> (-4.8046, -1.4989)
  line L98 (-4.8046, -1.4989) -> (-4, 0.0075)
  line L99 (-56.8409, 0) -> (-51.1995, -6.8437)
  line L100 (-51.1995, -6.8437) -> (-45.3544, 0)
  line L101 (-45.3544, 0) -> (-51.1995, 6.8437)
  line L102 (-51.1995, 6.8437) -> (-56.8409, 0)
  line L103 (-59.3235, 0) -> (-60.0719, 1.3)
  line L104 (-60.0719, 1.3) -> (-89.0719, 1.3)
  line L105 (-89.0719, 1.3) -> (-97.0393, 5.9)
  line L106 (-97.0393, 5.9) -> (-103.3231, 1.5)
  line L107 (-103.3231, 1.5) -> (-103.3231, -1.5)
  line L108 (-103.3231, -1.5) -> (-97.0393, -5.9)
  line L109 (-97.0393, -5.9) -> (-89.0719, -1.3)
  line L110 (-89.0719, -1.3) -> (-60.0719, -1.3)
  line L111 (-60.0719, -1.3) -> (-59.3235, 0)
  line L112 (-1.9935, 3.4678) -> (-1.0859, 4.9144)
  line L113 (-1.0859, 4.9144) -> (-2.4343, 6.3915)
  line L114 (-2.4343, 6.3915) -> (-20.127, 37.1684)
  line L115 (-20.127, 37.1684) -> (-21.9909, 36.0969)
  line L116 (-21.9909, 36.0969) -> (-4.2982, 5.32)
  line L117 (-4.2982, 5.32) -> (-3.7004, 3.4114)
  line L118 (-3.7004, 3.4114) -> (-1.9935, 3.4678)
  line L119 (-28.4205, 49.2257) -> (-31.5265, 40.9182)
  line L120 (-31.5265, 40.9182) -> (-22.6772, 39.2781)
  line L121 (-22.6772, 39.2781) -> (-19.673, 47.7619)
  line L122 (-19.673, 47.7619) -> (-28.4205, 49.2257)
  line L123 (-29.6618, 51.3757) -> (-28.9101, 52.6738)
  line L124 (-28.9101, 52.6738) -> (-43.4101, 77.7885)
  line L125 (-43.4101, 77.7885) -> (-43.4101, 86.9885)
  line L126 (-43.4101, 86.9885) -> (-50.3625, 90.2305)
  line L127 (-50.3625, 90.2305) -> (-52.9606, 88.7305)
  line L128 (-52.9606, 88.7305) -> (-53.6292, 81.0885)
  line L129 (-53.6292, 81.0885) -> (-45.6618, 76.4885)
  line L130 (-45.6618, 76.4885) -> (-31.1618, 51.3738)
  line L131 (-31.1618, 51.3738) -> (-29.6618, 51.3757)
  line L132 (2.0065, 3.4604) -> (3.7131, 3.3976)
  line L133 (3.7131, 3.3976) -> (4.318, 5.3039)
  line L134 (4.318, 5.3039) -> (22.1253, 36.0147)
  line L135 (22.1253, 36.0147) -> (20.2654, 37.0931)
  line L136 (20.2654, 37.0931) -> (2.4581, 6.3824)
  line L137 (2.4581, 6.3824) -> (1.1042, 4.9103)
  line L138 (1.1042, 4.9103) -> (2.0065, 3.4604)
  line L139 (28.4205, 49.2257) -> (19.673, 47.7619)
  line L140 (19.673, 47.7619) -> (22.6772, 39.2781)
  line L141 (22.6772, 39.2781) -> (31.5265, 40.9182)
  line L142 (31.5265, 40.9182) -> (28.4205, 49.2257)
  line L143 (29.6618, 51.3757) -> (31.1618, 51.3738)
  line L144 (31.1618, 51.3738) -> (45.6618, 76.4885)
  line L145 (45.6618, 76.4885) -> (53.6292, 81.0885)
  line L146 (53.6292, 81.0885) -> (52.9606, 88.7305)
  line L147 (52.9606, 88.7305) -> (50.3625, 90.2305)
  line L148 (50.3625, 90.2305) -> (43.4101, 86.9885)
  line L149 (43.4101, 86.9885) -> (43.4101, 77.7885)
  line L150 (43.4101, 77.7885) -> (28.9101, 52.6738)
  line L151 (28.9101, 52.6738) -> (29.6618, 51.3757)
  line L152 (59.3235, 0) -> (60.0719, -1.3)
  line L153 (60.0719, -1.3) -> (89.0719, -1.3)
  line L154 (89.0719, -1.3) -> (97.0393, -5.9)
  line L155 (97.0393, -5.9) -> (103.3231, -1.5)
  line L156 (103.3231, -1.5) -> (103.3231, 1.5)
  line L157 (103.3231, 1.5) -> (97.0393, 5.9)
  line L158 (97.0393, 5.9) -> (89.0719, 1.3)
  line L159 (89.0719, 1.3) -> (60.0719, 1.3)
  line L160 (60.0719, 1.3) -> (59.3235, 0)
  line L161 (56.8409, 0) -> (51.1995, 6.8437)
  line L162 (51.1995, 6.8437) -> (45.3544, 0)
  line L163 (45.3544, 0) -> (51.1995, -6.8437)
  line L164 (51.1995, -6.8437) -> (56.8409, 0)
  line L165 (4, -0.0075) -> (4.7989, -1.5168)
  line L166 (4.7989, -1.5168) -> (6.7523, -1.0876)
  line L167 (6.7523, -1.0876) -> (42.2523, -1.1537)
  line L168 (42.2523, -1.1537) -> (42.2563, 0.9962)
  line L169 (42.2563, 0.9962) -> (6.7563, 1.0624)
  line L170 (6.7563, 1.0624) -> (4.8046, 1.4989)
  line L171 (4.8046, 1.4989) -> (4, -0.0075)
  line L172 (29.6618, -51.3757) -> (28.9101, -52.6738)
  line L173 (28.9101, -52.6738) -> (43.4101, -77.7885)
  line L174 (43.4101, -77.7885) -> (43.4101, -86.9885)
  line L175 (43.4101, -86.9885) -> (50.3625, -90.2305)
  line L176 (50.3625, -90.2305) -> (52.9606, -88.7305)
  line L177 (52.9606, -88.7305) -> (53.6292, -81.0885)
  line L178 (53.6292, -81.0885) -> (45.6618, -76.4885)
  line L179 (45.6618, -76.4885) -> (31.1618, -51.3738)
  line L180 (31.1618, -51.3738) -> (29.6618, -51.3757)
  line L181 (28.4205, -49.2257) -> (31.5265, -40.9182)
  line L182 (31.5265, -40.9182) -> (22.6772, -39.2781)
  line L183 (22.6772, -39.2781) -> (19.673, -47.7619)
  line L184 (19.673, -47.7619) -> (28.4205, -49.2257)
  line L185 (1.9935, -3.4678) -> (1.0859, -4.9144)
  line L186 (1.0859, -4.9144) -> (2.4343, -6.3915)
  line L187 (2.4343, -6.3915) -> (20.127, -37.1684)
  line L188 (20.127, -37.1684) -> (21.9909, -36.0969)
  line L189 (21.9909, -36.0969) -> (4.2982, -5.32)
  line L190 (4.2982, -5.32) -> (3.7004, -3.4114)
  line L191 (3.7004, -3.4114) -> (1.9935, -3.4678)
  line L192 (-29.6618, -51.3757) -> (-31.1618, -51.3738)
  line L193 (-31.1618, -51.3738) -> (-45.6618, -76.4885)
  line L194 (-45.6618, -76.4885) -> (-53.6292, -81.0885)
  line L195 (-53.6292, -81.0885) -> (-52.9606, -88.7305)
  line L196 (-52.9606, -88.7305) -> (-50.3625, -90.2305)
  line L197 (-50.3625, -90.2305) -> (-43.4101, -86.9885)
  line L198 (-43.4101, -86.9885) -> (-43.4101, -77.7885)
  line L199 (-43.4101, -77.7885) -> (-28.9101, -52.6738)
  line L200 (-28.9101, -52.6738) -> (-29.6618, -51.3757)
  line L201 (-28.4205, -49.2257) -> (-19.673, -47.7619)
  line L202 (-19.673, -47.7619) -> (-22.6772, -39.2781)
  line L203 (-22.6772, -39.2781) -> (-31.5265, -40.9182)
  line L204 (-31.5265, -40.9182) -> (-28.4205, -49.2257)
  line L205 (-2.0065, -3.4604) -> (-3.7131, -3.3976)
  line L206 (-3.7131, -3.3976) -> (-4.318, -5.3039)
  line L207 (-4.318, -5.3039) -> (-22.1253, -36.0147)
  line L208 (-22.1253, -36.0147) -> (-20.2654, -37.0931)
  line L209 (-20.2654, -37.0931) -> (-2.4581, -6.3824)
  line L210 (-2.4581, -6.3824) -> (-1.1042, -4.9103)
  line L211 (-1.1042, -4.9103) -> (-2.0065, -3.4604)
  line L212 (-3.3169, 1.9233) -> (-2.3011, 0.0043)
  line L213 (-2.3011, 0.0043) -> (-3.324, -1.9109)
  line L214 (-3.324, -1.9109) -> (-1.1543, -1.9907)
  line L215 (-1.1543, -1.9907) -> (-0.0071, -3.8341)
  line L216 (-0.0071, -3.8341) -> (1.1469, -1.995)
  line L217 (1.1469, -1.995) -> (3.3169, -1.9233)
  line L218 (3.3169, -1.9233) -> (2.3011, -0.0043)
  line L219 (2.3011, -0.0043) -> (3.324, 1.9109)
  line L220 (3.324, 1.9109) -> (1.1543, 1.9907)
  line L221 (1.1543, 1.9907) -> (0.0071, 3.8341)
  line L222 (0.0071, 3.8341) -> (-1.1469, 1.995)
  line L223 (-1.1469, 1.995) -> (-3.3169, 1.9233)
  dimension "d452" = -1.5
extrude "Extrude7" add sketch "Sketch7" along normal up to surface (5 mm away) separate body contours L0 L6 L17 L26 | L2 L4 L17 L26 makes body 32 at (-10.5478, 60.4078, 1.6667) makes body 33 at (9.5982, 55.4737, 1.6667)
pattern_circular "C-Pattern6" count 6 over 360 about axis through (0, 0, 1.75) along (0, 0, 1) of bodies 32 33 makes body 34 at (-57.5885, 21.0693, 1.6667) makes body 35 at (-47.0408, -39.3385, 1.6667) makes body 36 at (10.5478, -60.4078, 1.6667) makes body 37 at (57.5885, -21.0693, 1.6667) makes body 38 at (47.0408, 39.3385, 1.6667) makes body 39 at (-43.2425, 36.0491, 1.6667) makes body 40 at (-52.8407, -19.4246, 1.6667) makes body 41 at (-9.5982, -55.4737, 1.6667) makes body 42 at (43.2425, -36.0491, 1.6667) makes body 43 at (52.8407, 19.4246, 1.6667)
combine "Combine2" operation add target body 19 tool bodies 32 33 34 35 36 37
combine "Combine3" operation add target body 38 tool bodies 43 19 39 40 41 42